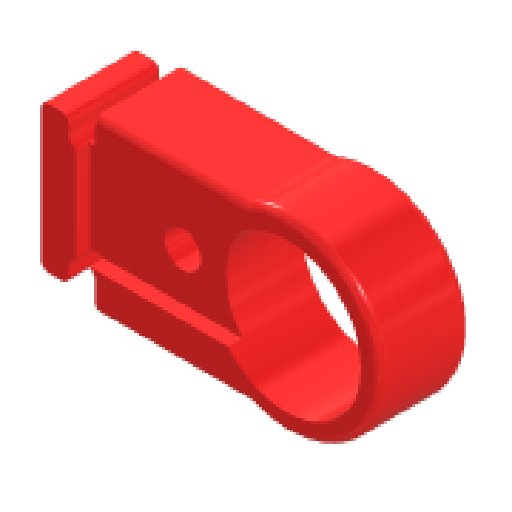
# Autodesk Inventor part: TransducerPCB_Holder
Saved by Autodesk Inventor 2023 (Build 270158000, 158)
## iProperties
Created: 2024-05-31
Part Number: TransducerPCB_Holder
Material: Generic
Document SubType Name: Modeling
Designer: Sven
Density: 1 g/cm^3
Appearance: Light Red
Author: Sven
Autodesk Inventor part; units mm, degrees
ref_plane "YZ Plane" through (0, 0, 0) normal (1, 0, 0) x (0, 1, 0)
ref_plane "XZ Plane" through (0, 0, 0) normal (0, 1, 0) x (-1, 0, 0)
ref_plane "XY Plane" through (0, 0, 0) normal (0, 0, 1) x (1, 0, 0)
sketch "Sketch1" plane through (0, 0, 0) normal (0, 0, 1) x (1, 0, 0)
  arc A0 (-13.7715, -6.45) -> (-16.2715, -6.45) centre (-15.0215, -6.45) ccw projected
  line L0 (-16.2715, -6.45) -> (-16.2715, -7.25) projected
  arc A1 (-17.2715, -8.25) -> (-16.2715, -7.25) centre (-17.2715, -7.25) ccw projected
  line L1 (-17.2715, -8.25) -> (-18.7715, -8.25) projected
  arc A2 (-19.7715, -7.25) -> (-18.7715, -8.25) centre (-18.7715, -7.25) ccw projected
  line L2 (-19.7715, -7.25) -> (-19.7715, 7.25) projected
  arc A3 (-18.7715, 8.25) -> (-19.7715, 7.25) centre (-18.7715, 7.25) ccw projected
  line L3 (-18.7715, 8.25) -> (-17.2715, 8.25) projected
  arc A4 (-16.2715, 7.25) -> (-17.2715, 8.25) centre (-17.2715, 7.25) ccw projected
  line L4 (-16.2715, 7.25) -> (-16.2715, 6.45) projected
  arc A5 (-16.2715, 6.45) -> (-13.7715, 6.45) centre (-15.0215, 6.45) ccw projected
  arc A6 (-13.5715, -6.45) -> (-16.4715, -6.45) centre (-15.0215, -6.45) ccw
  line L5 (-16.4715, -6.45) -> (-16.4715, -7.25)
  arc A7 (-17.2715, -8.05) -> (-16.4715, -7.25) centre (-17.2715, -7.25) ccw
  line L6 (-17.2715, -8.05) -> (-18.7715, -8.05)
  arc A8 (-19.5715, -7.25) -> (-18.7715, -8.05) centre (-18.7715, -7.25) ccw
  line L7 (-19.5715, -7.25) -> (-19.5715, 7.25)
  arc A9 (-18.7715, 8.05) -> (-19.5715, 7.25) centre (-18.7715, 7.25) ccw
  line L8 (-18.7715, 8.05) -> (-17.2715, 8.05)
  arc A10 (-16.4715, 7.25) -> (-17.2715, 8.05) centre (-17.2715, 7.25) ccw
  line L9 (-16.4715, 7.25) -> (-16.4715, 6.45)
  arc A11 (-16.4715, 6.45) -> (-13.5715, 6.45) centre (-15.0215, 6.45) ccw
  circle A12 centre (-5.5215, 0) radius 1.6 projected
  circle A13 centre (7.4785, 5) radius 0.5969 projected
  circle A14 centre (7.4785, -5) radius 0.5969 projected
  line L10 (13.4965, -5.336) -> (13.0086, -5.8402) projected
  arc A15 (13.4965, -5.336) -> (1.4605, 5.336) centre (7.4785, 0) ccw projected
  line L11 (1.1785, 5) -> (1.4605, 5.336) projected
  line L12 (-15.5215, 5) -> (1.1785, 5) projected
  line L13 (-15.5215, -5) -> (-15.5215, 5) projected
  line L14 (1.1785, -5) -> (-15.5215, -5) projected
  arc A16 (1.1785, -5) -> (13.0086, -5.8402) centre (7.4785, 0) ccw projected
  arc A17 (-0.6485, -6.45) -> (-0.6486, 6.45) centre (7.4785, 0) ccw
  line L15 (-0.6485, -6.45) -> (-15.5215, -6.45)
  line L16 (-15.5215, -6.45) -> (-15.5215, 6.45)
  line L17 (-15.5215, 6.45) -> (-0.6486, 6.45)
  line L18 (7.4785, 0) -> (-0.6485, -6.45)
  line L19 (7.4785, 0) -> (-0.6486, 6.45)
  circle A18 centre (7.4785, 0) radius 8.243
  point P0 (0, 0)
  point P1 (-15.03, 5)
  point P2 (-15.5215, 5.0889)
  point P3 (-13.5715, 6.45)
  dimension "d0" = 0.2
  dimension "d1" = 0.2
  constraints: 20 end point, 14 point on circle, 8 centre point, 3 point on line, 2 collinear, 2 parallel, 2 perpendicular, 1 coincident, 1 concentric, 1 horizontal, 10 other
  measures "d0" radial gap between concentric circles of A0 A6
  measures "d1" radial gap between concentric circles of A16 A18
extrude "Extrusion1" add sketch "Sketch1" against normal blind 10 contours A6 L14 A18 L18 L15 | L16 L14 A6 | A6 L5 A7 L6 A8 L7 A9 L8 A10 L9 A11 L16 L13 | L14 L13 L12 A18 | L18 A18 L19 A17 | L19 A18 L12 A11 L17 | A12
sketch "Sketch2" plane through (0, 0, 0) normal (0, 0, 1) x (1, 0, 0)
  circle A0 centre (-5.5215, 0) radius 1.6 projected
  circle A1 centre (7.4785, 5) radius 0.5969 projected
  circle A2 centre (7.4785, -5) radius 0.5969 projected
  line L0 (13.4965, -5.336) -> (13.0086, -5.8402) projected
  arc A3 (13.4965, -5.336) -> (1.4605, 5.336) centre (7.4785, 0) ccw projected
  line L1 (1.1785, 5) -> (1.4605, 5.336) projected
  line L2 (-15.5215, 5) -> (1.1785, 5) projected
  line L3 (-15.5215, -5) -> (-15.5215, 5) projected
  line L4 (1.1785, -5) -> (-15.5215, -5) projected
  arc A4 (1.1785, -5) -> (13.0086, -5.8402) centre (7.4785, 0) ccw projected
  line L5 (-15.7215, 5.2) -> (1.0853, 5.2)
  line L6 (1.0853, 5.2) -> (1.309, 5.4667)
  arc A5 (13.6433, -5.472) -> (1.309, 5.4667) centre (7.4785, 0) ccw
  line L7 (13.6433, -5.472) -> (13.1493, -5.9824)
  arc A6 (1.0826, -5.2) -> (13.1493, -5.9824) centre (7.4785, 0) ccw
  line L8 (1.0826, -5.2) -> (-15.7215, -5.2)
  line L9 (-15.7215, -5.2) -> (-15.7215, 5.2)
  point P0 (0, 0)
  dimension "d4" = 0.2
  constraints: 10 end point, 4 point on circle, 2 centre point, 6 other
  measures "d4" distance between parallel lines of L3 L9
extrude "Extrusion2" cut sketch "Sketch2" against normal blind 1.6 contours L0 A4 L4 L3 L2 L1 A3 | L5 L6 A5 L7 A6 L8 L9
sketch "Sketch3" plane through (-5.5215, 0, 0) normal (0, 0, 1) x (1, 0, 0)
  circle A0 centre (0, 0) radius 2
  point P0 (5.5215, 0)
  dimension "d7" = 4
  constraints: 1 centre point
  measures "d7" diameter of A0
extrude "Extrusion3" cut sketch "Sketch3" against normal blind 8
sketch "Sketch4" plane through (-19.5715, -7.25, 0) normal (-1, 0, 0) x (0, 0, 1)
  circle A0 centre (-5, 7.25) radius 2
  point P0 (0, 7.25)
  dimension "d10" = 4
  dimension "d11" = 5
  constraints: 1 centre point, 1 horizontal alignment
  measures "d10" diameter of A0
  measures "d11" distance of point (0, 7.25) A0.centre
extrude "Extrusion4" cut sketch "Sketch4" against normal blind 8
sketch "Sketch5" plane through (0, 0, 0) normal (0, 0, 1) x (1, 0, 0)
  line L0 (-13.7715, -9.5) -> (-13.7715, -6.45) projected
  line L1 (-13.7715, 6.45) -> (-13.7715, 9.5) projected
  line L2 (-13.7715, -9.5) -> (3.307, -9.5)
  arc A0 (-0.6485, -6.45) -> (-0.6486, 6.45) centre (7.4785, 0) ccw projected
  line L3 (-13.7715, 9.5) -> (3.307, 9.5)
  line L4 (-0.6485, -6.45) -> (-13.5715, -6.45) projected
  line L5 (-13.5715, -6.45) -> (-13.5715, -9.5)
  arc A1 (-15.03, 5) -> (-13.5715, 6.45) centre (-15.0215, 6.45) ccw projected
  line L6 (-13.5715, 6.45) -> (-13.5715, 9.5)
  line L7 (-0.6486, 6.45) -> (-13.5715, 6.45) projected
  point P0 (0, 0)
  constraints: 8 end point, 3 point on line, 2 horizontal, 2 point on circle, 1 perpendicular
extrude "Extrusion5" add sketch "Sketch5" against normal up to surface (10 mm away)
fillet "Fillet2" radius 1 6 edges at (17.854, 0, 0) (-5.1322, -9.5, 0) (-5.1323, 9.5, 0) (17.854, 0, -10) (-5.1323, 9.5, -10) (-5.1322, -9.5, -10)
body "Solid1"
